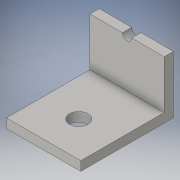
# Autodesk Inventor part: Angle Bracket for Bevel Gearbox
Saved by Autodesk Inventor 2016 (Build 200138000, 138)
## iProperties
Created: 2015-06-14
Part Number: Angle Bracket for Bevel Gearbox
Material: Generic
Document SubType Name: Modeling
Designer: steele
Density: 1 g/cm^3
Appearance: Default
Author: steele
Autodesk Inventor part; units mm, degrees
ref_plane "YZ Plane" through (0, 0, 0) normal (1, 0, 0) x (0, 1, 0)
ref_plane "XZ Plane" through (0, 0, 0) normal (0, 1, 0) x (-1, 0, 0)
ref_plane "XY Plane" through (0, 0, 0) normal (0, 0, 1) x (1, 0, 0)
sketch "Sketch1" plane through (0, 0, 0) normal (1, 0, 0) x (0, 1, 0)
  line L0 (0, 0) -> (39.4462, 0)
  line L1 (39.4462, 0) -> (39.4462, 6.35)
  line L2 (39.4462, 6.35) -> (6.35, 6.35)
  line L3 (6.35, 6.35) -> (6.35, 63.5)
  line L4 (6.35, 63.5) -> (0, 63.5)
  line L5 (0, 63.5) -> (0, 0)
  dimension "d0" = 6.35
  dimension "d1" = 6.35
  dimension "d4" = 33.0962
  dimension "d11" = 63.5
  constraints: 12 end point, 5 perpendicular, 1 horizontal
  measures "d0" distance of L3.end L4.end
  measures "d1" distance of L0.end L1.end
  measures "d4" distance between parallel lines of L3 L1
  measures "d11" distance between parallel lines of L0 L4
extrude "Extrusion1" add sketch "Sketch1" along normal mid plane 50.8
sketch "Sketch2" plane through (25.4, 39.4462, 0) normal (0, 0, -1) x (-1, 0, 0)
  line L0 (50.8, 0) -> (0, 0) projected
  arc A0 (22.225, 0) -> (28.575, 0) centre (25.4, 0) ccw
  line L1 (28.575, 0) -> (22.225, 0)
  point P0 (25.4, -39.4462)
  dimension "d5" = 6.35
  constraints: 2 end point, 2 point on circle, 2 point on line, 1 centre point, 1 midpoint
  measures "d5" diameter of A0
extrude "Extrusion2" cut sketch "Sketch2" against normal through all
sketch "Sketch4" plane through (-25.4, 0, 0) normal (0, -1, 0) x (1, 0, 0)
  line L0 (25.4, 0) -> (25.4, 63.5) construction
  line L1 (0, 63.5) -> (50.8, 63.5) construction
  line L2 (0, 39.4462) -> (50.8, 39.4462) construction
  line L3 (50.8, 0) -> (0, 0) construction
  circle A0 centre (25.4, 39.4462) radius 6.35
  dimension "d12" = 39.4462
  dimension "d13" = 12.7
  constraints: 4 end point, 2 midpoint, 1 centre point, 1 horizontal
  measures "d12" distance between parallel lines of L2 L3
  measures "d13" diameter of A0
extrude "Extrusion4" cut sketch "Sketch4" against normal through all
body "Solid1"
